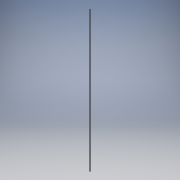
# Autodesk Inventor part: M6SS
Saved by Autodesk Inventor 2016 (Build 200138000, 138)
## iProperties
Created: 2017-07-13
Part Number: M6SS
Material: Steel
Document SubType Name: Modeling
Designer: ludwi
Density: 7.85 g/cm^3
Appearance: Plate
Mass: 226.393 g
Surface Area: 192.831 cm^2
Volume: 28.8398 cm^3
Author: ludwi
Autodesk Inventor part; units mm, degrees
ref_plane "YZ Plane" through (0, 0, 0) normal (1, 0, 0) x (0, 1, 0)
ref_plane "Work Plane1" through (2.1516, -2.5028, 640) normal (0, 0, 1) x (0.7481, -0.6636, 0)
ref_plane "Work Plane2" through (0.4379, 0.7784, 1020) normal (0, 0, 1) x (0.7481, -0.6636, 0)
sketch "Sketch1" plane through (0, 0, 0) normal (0, 0, 1) x (1, 0, 0)
  circle A0 centre (0, 0) radius 3
  dimension "d0" = 6
  constraints: 1 centre point, 1 coincident
  measures "d0" diameter of A0
extrude "Extrusion1" add sketch "Sketch1" along normal up to surface (1020 mm away)
thread "Thread1" size "M6x1" class "6g" standard "ANSI Metric M Profile" full length
body "Solid1"
